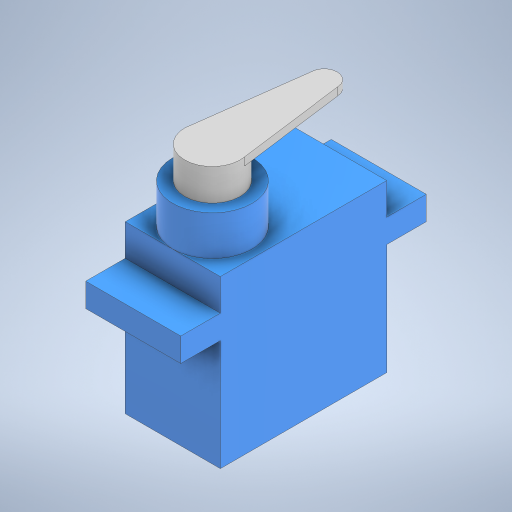
# Autodesk Inventor part: serwo
Saved by Autodesk Inventor 2023 (Build 270158000, 158)
## iProperties
Created: 2024-02-01
Part Number: serwo
Material: Ogólny
Document SubType Name: Modeling
Designer: domin
Density: 1 g/cm^3
Appearance: Domyślna
Author: domin
Autodesk Inventor part; units mm, degrees
ref_plane "YZ Plane" through (0, 0, 0) normal (1, 0, 0) x (0, 1, 0)
ref_plane "XZ Plane" through (0, 0, 0) normal (0, 1, 0) x (-1, 0, 0)
ref_plane "XY Plane" through (0, 0, 0) normal (0, 0, 1) x (1, 0, 0)
sketch "Szkic1" plane through (0, 0, 0) normal (0, 0, 1) x (1, 0, 0)
  line L0 (0, 0) -> (12, 0)
  line L1 (12, 0) -> (12, 21)
  line L2 (12, 21) -> (0, 21)
  line L3 (0, 21) -> (0, 0)
  dimension "d0" = 12
  dimension "d1" = 21
  constraints: 8 end point, 3 perpendicular, 1 horizontal
  measures "d0" distance of L0.start L0.end
  measures "d1" distance of L0.end L1.end
extrude "Wyciągnięcie proste1" add sketch "Szkic1" along normal blind 21
sketch "Szkic2" plane through (0, 0, 21) normal (0, 0, 1) x (1, 0, 0)
  line L0 (12, 0) -> (12, 21) projected
  line L1 (0, 17) -> (12, 17)
  line L2 (12, 17) -> (12, 14)
  line L3 (12, 14) -> (0, 14)
  line L4 (0, 14) -> (0, 17)
  line L5 (0, 17) -> (0, 14)
  line L6 (0, 21) -> (0, 0) projected
  dimension "d4" = 17
  dimension "d5" = 3
  dimension "d6" = 12
  constraints: 10 end point, 2 point on line, 1 collinear, 1 parallel, 1 perpendicular
  measures "d4" distance of L6.end L1.start
  measures "d5" distance of L1.end L2.end
  measures "d6" distance between parallel lines of L5 L0
extrude "Wyciągnięcie proste2" add sketch "Szkic2" along normal blind 5
sketch "Szkic3" plane through (0, 0, 0) normal (0, 0, -1) x (-1, 0, 0)
  line L0 (0, 17) -> (0, 14) projected
  line L1 (-12, 14) -> (0, 14)
  line L2 (0, 14) -> (0, 17)
  line L3 (0, 17) -> (-12, 17) projected
  line L4 (0, 17) -> (-12, 17)
  line L5 (-12, 14) -> (-12, 17) projected
  line L6 (-12, 17) -> (-12, 14)
  point P0 (0, 0)
  point P1 (-12, 0)
  constraints: 8 end point, 2 perpendicular, 1 collinear
extrude "Wyciągnięcie proste3" add sketch "Szkic3" along normal blind 5
sketch "Szkic4" plane through (0, 21, 0) normal (0, 1, 0) x (1, 0, 0)
  line L0 (12, -21) -> (0, -21) projected
  circle A0 centre (6, -16) radius 5
  point P0 (0, 0)
  dimension "d12" = 10
  dimension "d13" = 7.8102
  constraints: 1 centre point, 1 tangent
  measures "d12" diameter of A0
  measures "d13" distance of L0.start A0.centre
extrude "Wyciągnięcie proste4" add sketch "Szkic4" along normal blind 5
sketch "Szkic5" plane through (6, 26, 16) normal (0, 1, 0) x (1, 0, 0)
  circle A0 centre (0, 0) radius 3.5
  point P0 (-6, 16)
  dimension "d16" = 7
  constraints: 1 centre point
  measures "d16" diameter of A0
extrude "Wyciągnięcie proste5" add sketch "Szkic5" along normal blind 4
sketch "Szkic6" plane through (6, 30, 16) normal (0, 1, 0) x (1, 0, 0)
  arc A0 (1.654, 14.1744) -> (-1.6556, 14.1022) centre (0, 14.1022) ccw
  line L0 (-1.6556, 14.1022) -> (-3.5, 0)
  circle A1 centre (0, 0) radius 3.5 projected
  line L1 (1.654, 14.1744) -> (3.5266, 0)
  point P0 (-6, 16)
  point P1 (-3.3823, 0.9001)
  point P2 (3.4448, 0.6189)
  dimension "d19" = 1.6556
  dimension "d20" = 14.977
  dimension "d21" = 3.4962
  dimension "d22" = 3.4704
  dimension "d23" = 7.349
  dimension "d24" = 6.9673
  dimension "d25" = 3.2723
  dimension "d26" = 1.6493
  constraints: 4 end point, 2 point on circle, 1 centre point, 2 other
  measures "d19" radius of A0
  measures "d20" angle of L1 L0
  measures "d21" distance from line of point (0, 0) L1
  measures "d22" distance from line of point (0, 0) L0
  measures "d23" distance from line of point (-6, 16) L1
  measures "d24" distance from line of L1.end L0
  measures "d25" distance from line of L1.start L0
  measures "d26" distance from line of A0.centre L1
extrude "Wyciągnięcie proste6" add sketch "Szkic6" against normal blind 1 contours L1 A1 L0 A0
